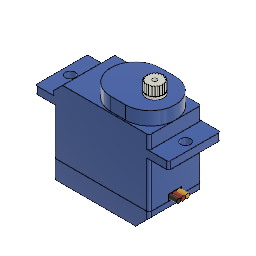
Servo Main Connector v2 (Autodesk Fusion 360 archive; units mm, degrees)
design "Servo"
Autodesk Fusion 360 part; units mm, degrees
sketch "bearing" plane through (0, 0, 0) normal (0, 0, 1) x (1, 0, 0)
  circle A0 centre (0, 0) radius 1.95
  circle A1 centre (0, 0) radius 0.5
  circle A2 centre (0, 0) radius 1.35
  dimension "d1" = 3.9
  dimension "d2" = 1
  dimension "d14" = 0.6
  measures "d1" diameter of A0
  measures "d2" diameter of A1
extrude "Extrude1" add sketch "bearing" along normal blind 0.6 contours A0 | A2 makes body 1
sketch "output spline" plane through (0, 0, 0) normal (0, 0, 1) x (1, 0, 0)
  line L0 (-0.75, 1.15) -> (0, 1.95)
  line L1 (0, 1.95) -> (0.75, 1.15)
  line L2 (0.75, 1.15) -> (-0.75, 1.15)
  line L3 (0, 1.95) -> (0, 1.15) construction
  line L4 (0, 1.15) -> (0, 0) construction
  dimension "d5" = 1.5
  dimension "d6" = 0.8
  dimension "d12" = 1.15
  measures "d5" distance of L0.start L1.end
  measures "d6" distance of L0.end L2
  measures "d12" distance of L3.end L4.end
extrude "Extrude2" add sketch "output spline" along normal blind 2 from surface at 0.6 bodies 1
pattern_circular "C-Pattern1" count 22 over 360 about axis through (0, 0, 0) along (0, 0, 1) of "Extrude2"
extrude "Extrude3" add sketch "bearing" along normal up to surface (2 mm away) from surface at 0.6 contours A2 bodies 1
sketch "base" plane through (0, 0, 0) normal (0, 0, 1) x (1, 0, 0)
  line L0 (-21.1, -5.9) -> (9, -5.9)
  line L1 (9, -5.9) -> (9, 5.9)
  line L2 (9, 5.9) -> (-21.1, 5.9)
  line L3 (-21.1, 5.9) -> (-21.1, -5.9)
  line L4 (-21.1, 0) -> (9, 0) construction
  line L5 (-6.05, -5.9) -> (-6.05, 5.9) construction
  line L6 (-1, 5.6) -> (-4.3, 5.6)
  arc A0 (-4.3, 5.6) -> (-4.3, -5.6) centre (-4.3, 0) ccw
  line L7 (-4.3, -5.6) -> (-1, -5.6)
  arc A1 (-1, -5.6) -> (-1, 5.6) centre (-1, 0) ccw
  line L8 (-1, 0) -> (-4.3, 0) construction
  circle A2 centre (6.95, 0) radius 1.1
  circle A3 centre (-19.05, 0) radius 1.1
  line L9 (-16.9, -5.9) -> (4.6, -5.9)
  line L10 (4.6, -5.9) -> (4.6, 5.9)
  line L11 (4.6, 5.9) -> (-16.9, 5.9)
  line L12 (-16.9, 5.9) -> (-16.9, -5.9)
  dimension "d18" = 11.8
  dimension "d19" = 30.1
  dimension "d20" = 9
  dimension "d21" = 11.2
  dimension "d22" = 3.3
  dimension "d24" = 4.4
  dimension "d25" = 2.2
  dimension "d26" = 2.05
  dimension "d27" = 2.2
  dimension "d28" = 26
  dimension "d29" = 21.5
  dimension "d30" = 11.8
  dimension "d31" = 4.2
  measures "d18" distance of L0.start L2.end
  measures "d19" distance of L1.end L2.end
  measures "d20" distance of origin L1
  measures "d21" diameter of A0
  measures "d22" distance of A1.centre A0.centre
  measures "d24" distance of L4.end A1
  measures "d25" diameter of A2
  measures "d26" distance of L4.end A2.centre
  measures "d27" diameter of A3
  measures "d28" distance of A2.centre A3.centre
  measures "d29" distance of L9.start L9.end
  measures "d30" distance of L9.start L11.end
  measures "d31" distance of L3 L12
extrude "Extrude4" add sketch "base" against normal blind 3 separate body contours L6 A0 L7 A1 makes body 2
extrude "Extrude5" add sketch "base" against normal blind 3 from surface at -3 contours L6 A0 L7 A1 | L0 L2 L9 L10 L11 L12 bodies 2
chamfer "Chamfer2" distance 2 angle 45 1 edges at (-16.9, 0, -3) on bodies 2
extrude "Extrude6" add sketch "base" against normal blind 1.7 from surface at -6 contours L0 L2 L3 L12 | L6 A0 L7 A1 | L0 L2 L9 L10 L11 L12 | L0 L1 L2 L10 bodies 2
extrude "Extrude7" add sketch "base" against normal blind 10.4 from surface at -7.7 contours L6 A0 L7 A1 | L0 L2 L9 L10 L11 L12 bodies 2
sketch "bottom cover" plane through (0, 0, -18.1) normal (0, 0, -1) x (1, 0, 0)
  line L0 (4.6, 5.9) -> (-16.9, 5.9)
  line L1 (-16.9, 5.9) -> (-16.9, -5.9)
  line L2 (-16.9, -5.9) -> (4.6, -5.9)
  line L3 (4.6, -5.9) -> (4.6, 5.9)
extrude "Extrude8" add sketch "bottom cover" along normal blind 4.2 separate body makes body 3
chamfer "Chamfer3" distance 3 angle 45 1 edges at (4.6, 0, -22.3) on bodies 3
fillet "Fillet1" radius 0.5 15 edges at (4.6, 5.9, -4.5) (4.6, -5.9, -4.5) (4.6, -5.9, -12.9) (4.6, 5.9, -12.9) (-16.9, 5.9, -5.5) (-16.9, 5.9, -12.9) (-16.9, -5.9, -12.9) (-21.1, 5.9, -6.85) (9, 5.9, -6.85) (-21.1, -5.9, -6.85) (9, -5.9, -6.85) (4.6, 5.9, -18.7) (4.6, -5.9, -18.7) (-16.9, 5.9, -20.2) (-16.9, -5.9, -20.2) on bodies 2 3
sketch "wire port" plane through (4.6, 0, 0) normal (1, 0, 0) x (0, -1, 0)
  line L0 (-1.5, 18.1) -> (1.5, 18.1)
  line L1 (1.5, 18.1) -> (1.5, 16.7)
  line L2 (1.5, 16.7) -> (-1.5, 16.7)
  line L3 (-1.5, 16.7) -> (-1.5, 18.1)
  circle A0 centre (-1, 17.4) radius 0.5
  circle A1 centre (0, 17.4) radius 0.5
  circle A2 centre (1, 17.4) radius 0.5
  line L4 (0, 17.4) -> (0, 16.7) construction
  line L5 (-5.4, 18.1) -> (-5.4, 7.7)
  line L6 (-5.4, 7.7) -> (5.4, 7.7)
  line L7 (5.4, 7.7) -> (5.4, 18.1)
  line L8 (5.4, 18.1) -> (-5.4, 18.1)
  dimension "d49" = 3
  dimension "d50" = 1.4
  dimension "d51" = 1
  dimension "d52" = 1
  dimension "d53" = 1
  dimension "d54" = 0.7
  dimension "d55" = 0.7
  dimension "d56" = 0.7
  dimension "d57" = 1
  dimension "d58" = 1
  measures "d49" distance of L0.start L0.end
  measures "d50" distance of L0.start L2.end
  measures "d51" diameter of A0
  measures "d52" diameter of A1
  measures "d53" diameter of A2
  measures "d54" distance of L0 A2.centre
  measures "d55" distance of L0 A1.centre
  measures "d56" distance of L0 A0.centre
  measures "d57" distance of A0.centre A1.centre
  measures "d58" distance of A1.centre A2.centre
extrude "Extrude9" cut sketch "wire port" against normal blind 0.2 contours L0 L1 L3 A0 A1 A2 L8 | L1 L2 L3 A0 A1 A2 | A0 | A2 | A1 bodies 2
extrude "Extrude10" add sketch "wire port" along normal blind 2 from surface at -0.2 separate body contours A2 makes body 4
extrude "Extrude11" add sketch "wire port" along normal blind 2 from surface at -0.2 separate body contours A1 makes body 5
extrude "Extrude12" add sketch "wire port" along normal blind 2 from surface at -0.2 separate body contours A0 makes body 6
equation "d57 = ( 3 / 3 ) * 1 mm"
equation "d58 = ( 3 / 3 ) * 1 mm"
named bodies: "output spline", "case", "bottom cover", "ground wire", "voltage wire", "signal wire"
